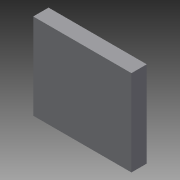
# Autodesk Inventor part: Place holder for wheels
Saved by Autodesk Inventor 2014 SP1 (Build 180222100, 222)
## iProperties
Created: 2014-01-20
Part Number: Place holder for wheels
Material: Generic
Document SubType Name: Modeling
Designer: habib asif
Density: 1 g/cm^3
Appearance: Default
Author: habib asif
Autodesk Inventor part; units mm, degrees
ref_plane "YZ Plane" through (0, 0, 0) normal (1, 0, 0) x (0, 1, 0)
ref_plane "XZ Plane" through (0, 0, 0) normal (0, 1, 0) x (-1, 0, 0)
ref_plane "XY Plane" through (0, 0, 0) normal (0, 0, 1) x (1, 0, 0)
sketch "Sketch1" plane through (0, 0, 0) normal (0, 0, 1) x (1, 0, 0)
  line L0 (-11.4652, 5.8606) -> (191.7348, 5.8606)
  line L1 (191.7348, 5.8606) -> (191.7348, -171.9394)
  line L2 (191.7348, -171.9394) -> (-11.4652, -171.9394)
  line L3 (-11.4652, -171.9394) -> (-11.4652, 5.8606)
  dimension "d0" = 203.2
  dimension "d1" = 177.8
  constraints: 8 end point, 2 parallel, 1 horizontal, 1 perpendicular
  measures "d0" distance of L1.end L2.end
  measures "d1" distance of L0.end L1.end
extrude "Extrusion1" add sketch "Sketch1" along normal blind 31.75
body "Solid1"
